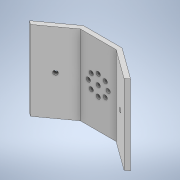
# Autodesk Inventor part: 10 bracket
Saved by Autodesk Inventor 2020 (Build 240168000, 168)
## iProperties
Created: 2020-02-18
Part Number: 10 bracket
Material: Generic
Document SubType Name: Modeling
Designer: Ball
Density: 1 g/cm^3
Appearance: Default
Author: Ball
Autodesk Inventor part; units mm, degrees
ref_plane "YZ Plane" through (0, 0, 0) normal (1, 0, 0) x (0, 1, 0)
ref_plane "XZ Plane" through (0, 0, 0) normal (0, 1, 0) x (-1, 0, 0)
ref_plane "XY Plane" through (0, 0, 0) normal (0, 0, 1) x (1, 0, 0)
sketch "Sketch1" plane through (0, 0, 0) normal (0, 1, 0) x (-1, 0, 0)
  line L0 (44.8336, -32.5735) -> (17.1249, -52.705)
  line L1 (17.1249, -52.705) -> (-17.1249, -52.705)
  line L2 (-17.1249, -52.705) -> (-44.8336, -32.5735)
  line L3 (48.4634, -35.2108) -> (18.5114, -56.9722)
  line L4 (18.5114, -56.9722) -> (-18.5114, -56.9722)
  line L5 (-18.5114, -56.9722) -> (-48.4634, -35.2108)
  line L6 (48.4634, -35.2108) -> (44.8336, -32.5735)
  line L7 (-44.8336, -32.5735) -> (-48.4634, -35.2108)
  point P0 (0, 0)
  point P1 (0, 0)
  point P2 (0, 0)
  dimension "d0" = 52.705
  dimension "d1" = 4.2672
  constraints: 16 end point, 2 coincident, 12 other
  measures "d0" distance from line of L1 point (0, 0)
  measures "d1" distance between parallel lines of L1 L4
extrude "Extrusion1" add sketch "Sketch1" along normal blind 76.2
sketch "Sketch2" plane through (18.5114, 0, -56.9722) normal (0.5877853, 0, -0.809017) x (-0.809017, 0, -0.5877853)
  circle A0 centre (-18.5114, 38.1) radius 2.032
  line L0 (-37.0228, 76.2) -> (0, 76.2) projected
  point P0 (-18.5114, 0)
  dimension "d4" = 4.064
  dimension "d5" = 38.1
  constraints: 1 centre point
  measures "d4" diameter of A0
  measures "d5" distance from line of L0 A0.centre
sketch "Sketch3" plane through (18.5114, 0, -56.9722) normal (0, 0, -1) x (-1, 0, 0)
  circle A0 centre (18.5114, 38.1) radius 2.032
  line L0 (0, 76.2) -> (37.0228, 76.2) projected
  point P0 (18.5114, 0)
  dimension "d6" = 4.064
  dimension "d7" = 38.1
  constraints: 1 centre point
  measures "d6" diameter of A0
  measures "d7" distance from line of L0 A0.centre
sketch "Sketch4" plane through (-48.4634, 0, -35.2108) normal (-0.5877853, 0, -0.809017) x (-0.809017, 0, 0.5877853)
  circle A0 centre (-18.5114, 38.1) radius 2.032
  line L0 (-37.0228, 76.2) -> (0, 76.2) projected
  point P0 (-18.5114, 0)
  dimension "d8" = 4.064
  dimension "d9" = 38.1
  constraints: 1 centre point
  measures "d8" diameter of A0
  measures "d9" distance from line of L0 A0.centre
extrude "Extrusion2" cut sketch "Sketch2" against normal through all
extrude "Extrusion3" cut sketch "Sketch3" against normal blind 4.2672
extrude "Extrusion4" cut sketch "Sketch4" against normal blind 4.2672
sketch "Sketch5" plane through (18.5114, 0, -56.9722) normal (0, 0, -1) x (-1, 0, 0)
  circle A0 centre (18.5114, 38.1) radius 2.032 projected
  circle A1 centre (18.5114, 47.5742) radius 2.032
  circle A2 centre (11.8121, 44.7993) radius 2.032
  circle A3 centre (9.0372, 38.1) radius 2.032
  circle A4 centre (11.8121, 31.4007) radius 2.032
  circle A5 centre (18.5114, 28.6258) radius 2.032
  circle A6 centre (25.2107, 31.4007) radius 2.032
  circle A7 centre (27.9856, 38.1) radius 2.032
  circle A8 centre (25.2107, 44.7993) radius 2.032
  point P0 (18.5114, 0)
  dimension "d17" = 4.064
  dimension "d21" = 360
  constraints: 8 centre point, 17 other
  measures "d17" diameter of A1
extrude "Extrusion5" cut sketch "Sketch5" against normal through all contours A1 | A2 | A3 | A4 | A5 | A6 | A7 | A8
body "Solid1"
